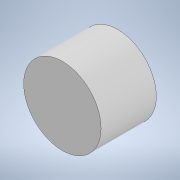
# Autodesk Inventor part: Корпус дифференциала
Saved by Autodesk Inventor 2020 (Build 240168000, 168)
## iProperties
Created: 2021-03-14
Part Number: Корпус дифференциала
Material: Типовые
Document SubType Name: Modeling
Designer: Антон
Density: 1 g/cm^3
Appearance: По умолчанию
Author: Антон
Autodesk Inventor part; units mm, degrees
ref_plane "YZ Plane" through (0, 0, 0) normal (1, 0, 0) x (0, 1, 0)
ref_plane "XZ Plane" through (0, 0, 0) normal (0, 1, 0) x (-1, 0, 0)
ref_plane "XY Plane" through (0, 0, 0) normal (0, 0, 1) x (1, 0, 0)
sketch "Эскиз1" plane through (0, 0, 0) normal (0, 0, 1) x (1, 0, 0)
  circle A0 centre (0, 0) radius 7
  dimension "d0" = 14
  constraints: 1 centre point, 1 coincident
  measures "d0" diameter of A0
extrude "Выдавливание1" add sketch "Эскиз1" along normal blind 10
sketch "Эскиз2" plane through (0, 0, 0) normal (0, 0, -1) x (-1, 0, 0)
  circle A0 centre (0, 0) radius 5
  circle A1 centre (0, 0) radius 7 projected
  line L0 (-3.5355, 3.5355) -> (3.5355, 3.5355)
  line L1 (3.5355, 3.5355) -> (3.5355, -3.5355)
  line L2 (3.5355, -3.5355) -> (-3.5355, -3.5355)
  line L3 (-3.5355, -3.5355) -> (-3.5355, 3.5355)
  line L4 (-3.5355, 3.5355) -> (3.5355, -3.5355) construction
  line L5 (3.5355, 3.5355) -> (-3.5355, -3.5355) construction
  circle A2 centre (3.5355, 3.5355) radius 2
  circle A3 centre (3.5355, -3.5355) radius 2
  circle A4 centre (-3.5355, 3.5355) radius 2
  circle A5 centre (-3.5355, -3.5355) radius 2
  point P0 (-1.8671, -4.6383)
  point P1 (1.8671, -4.6383)
  point P2 (4.6383, -1.8671)
  point P3 (4.6383, 1.8671)
  point P4 (1.8671, 4.6383)
  point P5 (-1.8671, 4.6383)
  point P6 (-4.6383, 1.8671)
  point P7 (-4.6383, -1.8671)
  dimension "d3" = 10
  dimension "d4" = 14
  dimension "d8" = 4
  dimension "d9" = 4
  dimension "d10" = 4
  dimension "d11" = 4
  constraints: 12 end point, 5 coincident, 4 centre point, 2 midpoint, 2 parallel, 2 perpendicular, 1 horizontal, 3 other
  measures "d4" diameter of A1
  measures "d8" diameter of A2
  measures "d9" diameter of A3
  measures "d10" diameter of A4
  measures "d11" diameter of A5
ref_plane "РабПлоскость1" through (0, 0, 6) normal (0, 0, 1) x (1, 0, 0)
extrude "Выдавливание2" cut sketch "Эскиз2" against normal up to surface (6 mm away) contours A0 A3 L1 A2 | L1 A3 L2 A5 L3 A4 L0 A2 | A2 L0 A4 A0 | A0 A5 L2 A3 | L3 A5 A0 A4
sketch "Эскиз3" plane through (0, 0, 0) normal (0, 0, -1) x (-1, 0, 0)
  arc A0 (1.8671, 4.6383) -> (4.6383, 1.8671) centre (3.5355, 3.5355) ccw projected
  arc A1 (4.6383, -1.8671) -> (1.8671, -4.6383) centre (3.5355, -3.5355) ccw projected
  arc A2 (-4.6383, 1.8671) -> (-1.8671, 4.6383) centre (-3.5355, 3.5355) ccw projected
  arc A3 (-1.8671, -4.6383) -> (-4.6383, -1.8671) centre (-3.5355, -3.5355) ccw projected
  point P0 (0, 0)
hole "Отверстие1" at (-3.5355, 3.5355, 0) at (3.5355, 3.5355, 0) at (3.5355, -3.5355, 0) at (-3.5355, -3.5355, 0) direction (0, 0, 1) diameter 2 depth 6 tip angle 118
equation "\"d9\" = d8"
equation "\"d10\" = d8"
equation "\"d11\" = d10"
